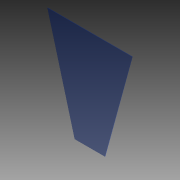
# Autodesk Inventor part: back window
Saved by Autodesk Inventor 2012 (Build 160160000, 160)
## iProperties
Created: 2011-12-02
Part Number: back window
Material: Polycarbonate, Clear
Document SubType Name: Modeling
Designer: Antonella
Mass: 163.461 g
Surface Area: 1735.65 cm^2
Volume: 136.217 cm^3
Density: 1.2 g/cm^3
Author: Antonella
Autodesk Inventor part; units mm, degrees
ref_plane "YZ Plane" through (0, 0, 0) normal (1, 0, 0) x (0, 1, 0)
ref_plane "XZ Plane" through (0, 0, 0) normal (0, 1, 0) x (-1, 0, 0)
ref_plane "XY Plane" through (0, 0, 0) normal (0, 0, 1) x (1, 0, 0)
sketch "Sketch1" plane through (0, 0, 0) normal (0, 0, 1) x (1, 0, 0)
  line L0 (-248.92, 0) -> (248.92, 0) projected
  line L1 (0, -83.82) -> (0, 502.92) projected
  line L2 (-177.8, 419.1) -> (177.8, 419.1)
  line L3 (177.8, 419.1) -> (63.5, 0)
  line L4 (63.5, 0) -> (-63.5, 0)
  line L5 (-63.5, 0) -> (-177.8, 419.1)
  point P0 (0, 0)
  point P1 (0, 419.1)
  dimension "d0" = 127
  dimension "d1" = 355.6
  dimension "d2" = 419.1
  constraints: 8 end point, 2 perpendicular, 1 collinear, 1 equal length, 1 midpoint, 1 vertical alignment
  measures "d0" distance of L3.end L4.end
  measures "d1" distance of L2.start L2.end
  measures "d2" distance between parallel lines of L2 L4
extrude "Extrusion1" add sketch "Sketch1" along normal blind 1.5875
body "Solid1"
